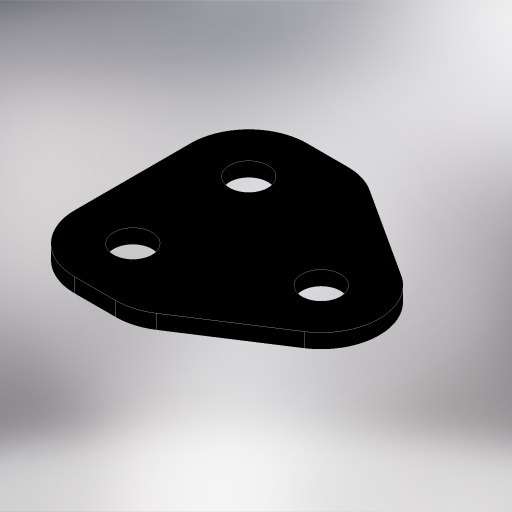
# Autodesk Inventor part: 742 2.1 Gusset A
Saved by Autodesk Inventor 2024 (Build 280153000, 153)
## iProperties
Created: 2023-10-21
Part Number: 742 2.1 Gusset A
Material: Generic
Document SubType Name: Modeling
Designer: aaron
Density: 1 g/cm^3
Appearance: Default
Author: aaron
Autodesk Inventor part; units mm, degrees
ref_plane "YZ Plane" through (0, 0, 0) normal (1, 0, 0) x (0, 1, 0)
ref_plane "XZ Plane" through (0, 0, 0) normal (0, 1, 0) x (-1, 0, 0)
ref_plane "XY Plane" through (0, 0, 0) normal (0, 0, 1) x (1, 0, 0)
sketch "Sketch1" plane through (0, 0, 0) normal (0, 1, 0) x (-1, 0, 0)
  line L0 (-6.35, -12.7) -> (6.35, -12.7)
  line L1 (6.35, -12.7) -> (6.35, 12.7)
  line L2 (6.35, 12.7) -> (-6.35, 12.7)
  line L3 (-6.35, 12.7) -> (-6.35, -12.7)
  line L4 (-6.35, -12.7) -> (6.35, 12.7) construction
  line L5 (6.35, -12.7) -> (-6.35, 12.7) construction
  circle A0 centre (0, 6.35) radius 2.1082
  circle A1 centre (0, -6.35) radius 2.1082
  circle A2 centre (-14.2875, 0) radius 2.1082
  circle A3 centre (-14.2875, 0) radius 6.35
  line L6 (-6.35, 12.7) -> (-17.7373, 5.3311)
  line L7 (-17.7373, -5.3311) -> (-6.35, -12.7)
  point P0 (0, 0)
  dimension "d0" = 25.4
  dimension "d1" = 12.7
  dimension "d2" = 4.2164
  dimension "d3" = 4.2164
  dimension "d4" = 6.35
  dimension "d5" = 6.35
  dimension "d6" = 6.35
  dimension "d7" = 4.2164
  dimension "d8" = 7.9375
  dimension "d9" = 12.7
  constraints: 16 end point, 4 centre point, 2 midpoint, 2 parallel, 2 point on circle, 2 tangent, 1 coincident, 1 horizontal, 1 perpendicular, 1 point on line
  measures "d0" distance between parallel lines of L2 L0
  measures "d1" distance between parallel lines of L3 L1
  measures "d2" diameter of A1
  measures "d3" diameter of A0
  measures "d4" distance from line of L2 A0.centre
  measures "d5" distance from line of L0 A1.centre
  measures "d6" distance from line of L1 A1.centre
  measures "d7" diameter of A2
  measures "d8" distance from line of A2.centre L3
  measures "d9" diameter of A3
extrude "Extrusion1" add sketch "Sketch1" along normal blind 1.5875
fillet "Fillet1" radius 6.35 4 edges at (6.35, 0.7937, 12.7) (-6.35, 0.7937, 12.7) (6.35, 0.7937, -12.7) (-6.35, 0.7937, -12.7)
body "Solid1"
